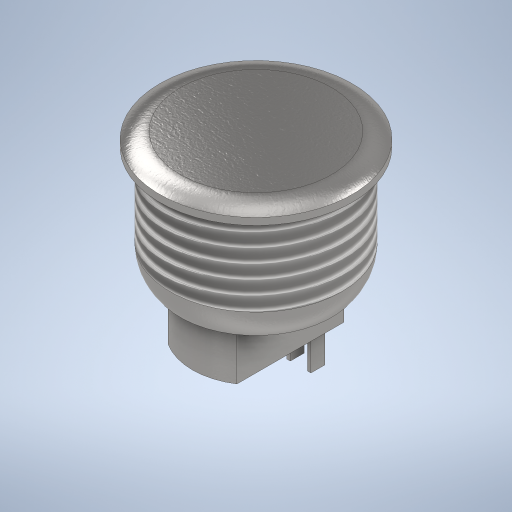
# Autodesk Inventor part: Druckknopf_Konsole_groß
Saved by Autodesk Inventor 2024 (Build 280153000, 153)
## iProperties
Created: 2024-05-02
Part Number: Druckknopf_Konsole_groß
Material: Stahl, galvanisiert
Document SubType Name: Modeling
Designer: haniv
Density: 7.85 g/cm^3
Appearance: Galvanisiert
Author: haniv
Autodesk Inventor part; units mm, degrees
ref_plane "YZ Plane" through (0, 0, 0) normal (1, 0, 0) x (0, 1, 0)
ref_plane "XZ Plane" through (0, 0, 0) normal (0, 1, 0) x (-1, 0, 0)
ref_plane "XY Plane" through (0, 0, 0) normal (0, 0, 1) x (1, 0, 0)
sketch "Skizze1" plane through (0, 0, 0) normal (0, 1, 0) x (-1, 0, 0)
  line L0 (0, 0) -> (0, -100) construction
  line L1 (0, 0) -> (11, 0)
  arc A0 (14, -1) -> (11, 0) centre (11, -5) ccw
  line L2 (14, -1) -> (14, -2)
  line L3 (14, -2) -> (12.5, -2)
  line L4 (12.5, -2) -> (12.5, -14)
  arc A1 (11, -18) -> (12.5, -14) centre (6.4167, -14) ccw
  line L5 (11, -18) -> (9.25, -18)
  line L6 (9.25, -18) -> (9.25, -25.5)
  line L7 (9.25, -25.5) -> (0, -25.5)
  line L8 (0, 0) -> (0, -25.5)
  point P0 (13.25, -2)
  dimension "d0" = 100
  dimension "d1" = 25
  dimension "d2" = 28
  dimension "d3" = 2
  dimension "d4" = 1
  dimension "d5" = 3
  dimension "d6" = 12
  dimension "d7" = 4
  dimension "d8" = 22
  dimension "d9" = 18.5
  dimension "d10" = 7.5
  constraints: 18 end point, 5 perpendicular, 4 point on circle, 3 vertical, 2 centre point, 2 tangent, 1 horizontal, 1 midpoint, 1 point on line
  measures "d0" distance of L0.start L0.end
  measures "d1" diameter of L4 L0
  measures "d2" diameter of L2 L0
  measures "d3" distance from line of L1 point (13.25, -2)
  measures "d4" distance from line of L1 L2.start
  measures "d5" distance from line of L2 L1.end
  measures "d6" distance of L3.end L4.end
  measures "d7" distance from line of L5 L4.end
  measures "d8" diameter of L5.start L0
  measures "d9" diameter of L6 L0
  measures "d10" distance of L5.end L6.end
revolve "Umdrehung1" add sketch "Skizze1" angle 360 about axis through (0, 0, 0) along (0, 0, -1)
thread "Gewinde1" size "M25x2" class "6g" standard "ISO Metric profile" full length
sketch "Skizze2" plane through (0, 0, -25.5) normal (0, 0, -1) x (-1, 0, 0)
  circle A0 centre (0, 0) radius 9.25 projected
  line L0 (5, 7.7822) -> (-5, 7.7822)
  line L1 (-5, 7.7822) -> (-5, -7.7822)
  line L2 (-5, -7.7822) -> (5, -7.7822)
  line L3 (5, -7.7822) -> (5, 7.7822)
  dimension "d14" = 10
  constraints: 8 end point, 3 point on circle, 2 parallel, 1 horizontal, 1 perpendicular
  measures "d14" distance between parallel lines of L1 L3
extrude "Extrusion1" cut sketch "Skizze2" against normal up to surface (7.5 mm away) contours A0 L3 | L1 A0
sketch "Skizze3" plane through (0, 0, -25.5) normal (0, 0, -1) x (-1, 0, 0)
  line L0 (3.5, 7) -> (3, 7)
  line L1 (3, 7) -> (3, 5)
  line L2 (3, 5) -> (3.5, 5)
  line L3 (3.5, 5) -> (3.5, 7)
  point P0 (0, 0)
  point P1 (3, 6)
  dimension "d17" = 0.5
  dimension "d18" = 2
  dimension "d19" = 5
  dimension "d20" = 3
  constraints: 8 end point, 2 parallel, 1 horizontal, 1 midpoint, 1 perpendicular
  measures "d17" distance of L1.end L2.end
  measures "d18" distance of L2.end L0.start
  measures "d19" distance from line of point (0, 0) L2
  measures "d20" horizontal distance of point (0, 0) point (3, 6)
extrude "Extrusion2" add sketch "Skizze3" along normal blind 6
pattern_linear "Rechteckige Anordnung1" count 3 spacing 3 along (1, 0, 0) of "Extrusion2"
